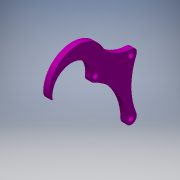
# Autodesk Inventor part: climb hook
Saved by Autodesk Inventor 2017 SP1 (Build 210196100, 196)
## iProperties
Created: 2018-03-18
Part Number: climb hook
Material: Aluminum 6061
Document SubType Name: Modeling
Designer: Ben
Density: 2.7 g/cm^3
Appearance: Magenta
Mass: 51.4695 g
Surface Area: 88.6391 cm^2
Volume: 19.0628 cm^3
Author: Ben
Autodesk Inventor part; units mm, degrees
ref_plane "YZ Plane" through (0, 0, 0) normal (1, 0, 0) x (0, 1, 0)
ref_plane "XZ Plane" through (0, 0, 0) normal (0, 1, 0) x (-1, 0, 0)
ref_plane "XY Plane" through (0, 0, 0) normal (0, 0, 1) x (1, 0, 0)
sketch "Sketch1" plane through (0, 0, 0) normal (1, 0, 0) x (0, 1, 0)
  line L0 (31.75, 0) -> (-31.75, 0) construction
  line L1 (-31.75, 0) -> (-31.75, -20.6375) construction
  line L2 (31.75, -20.6375) -> (31.75, 20.6375) construction
  circle A0 centre (31.75, -20.6375) radius 3.175
  circle A1 centre (31.75, 20.6375) radius 3.175
  circle A2 centre (-31.75, -20.6375) radius 3.175
  arc A3 (32.8083, 26.8987) -> (31.75, 70.5216) centre (36.5125, 48.8128) ccw
  arc A4 (32.8083, 26.8987) -> (25.9468, 23.2154) centre (31.75, 20.6375) ccw
  arc A5 (-31.75, -14.2875) -> (-29.3077, -26.499) centre (-31.75, -20.6375) ccw
  arc A6 (-31.75, -14.2875) -> (25.9468, 23.2154) centre (-31.75, 48.8462) ccw
  arc A7 (29.3077, -26.499) -> (38.0929, -20.9379) centre (31.75, -20.6375) ccw
  arc A8 (29.3077, -26.499) -> (-29.3077, -26.499) centre (0, -96.8375) ccw
  circle A9 centre (42.8625, 48.8128) radius 15.875 construction
  line L3 (42.8625, 48.8128) -> (36.5125, 48.8128) construction
  arc A10 (40.1665, 75.3383) -> (31.75, 70.5216) centre (40.0305, 65.8143) ccw
  arc A11 (53.499, 11.1952) -> (40.1665, 75.3383) centre (39.6875, 41.7816) ccw
  line L4 (40.0305, 65.8143) -> (41.016, 70.5768) construction
  line L5 (53.499, 11.1952) -> (45.6591, 28.5572) construction
  line L6 (39.6875, 41.7816) -> (39.6875, 48.8128) construction
  arc A12 (53.499, 11.1952) -> (38.0929, -20.9379) centre (83.8247, -23.1041) ccw
  line L7 (34.1811, 18.5954) -> (48.768, 6.3428) construction
  line L8 (-16.226, -22.3851) -> (-18.3063, -12.8396) construction
  line L9 (31.75, -20.6375) -> (-31.75, -20.6375) construction
  point P0 (0, 0)
  point P1 (0, 0)
  dimension "d0" = 63.5
  dimension "d1" = 41.275
  dimension "d2" = 6.35
  dimension "d4" = 6.35
  dimension "d6" = 44.45
  dimension "d7" = 31.75
  dimension "d8" = 4.7625
  dimension "d9" = 9.525
  dimension "d10" = 4.7625
  dimension "d12" = 19.05
  dimension "d13" = 19.05
  dimension "d19" = 9.7696
  constraints: 23 point on circle, 20 end point, 12 centre point, 9 tangent, 7 coincident, 6 line through centre, 3 equal radius, 3 horizontal, 3 midpoint, 2 point on line, 2 vertical, 1 perpendicular, 5 other
  measures "d0" distance of L0.start L0.end
  measures "d1" distance of L2.start L2.end
  measures "d2" diameter of A0
  measures "d4" radius of A4
  measures "d6" diameter of A3
  measures "d7" diameter of A9
  measures "d8" distance from line of L2 L3.end
  measures "d9" radius of A10
  measures "d10" vertical distance of L4.start L4.end
  measures "d12" distance of L5.start L5.end
  measures "d13" distance of L7.start L7.end
  measures "d19" distance of L8.start L8.end
extrude "Extrusion1" add sketch "Sketch1" along normal blind 6.35
fillet "Fillet1" radius 25.4 1 edges at (3.175, 53.499, 11.1952)
fillet "Fillet1" radius 0.508 1 edges at (3.175, 31.75, 70.5216)
equation "\"d10\" = 0.5 * d9"
body "Solid1"
